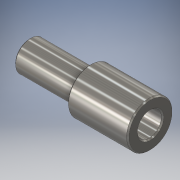
# Autodesk Inventor part: Motor-Adapter
Saved by Autodesk Inventor 2016 (Build 200138000, 138)
## iProperties
Created: 2015-05-19
Part Number: Motor-Adapter
Material: Generic
Document SubType Name: Modeling
Designer: jonathan
Density: 1 g/cm^3
Appearance: Steel - Polished
Mass: 1.0291 g
Surface Area: 9.66443 cm^2
Volume: 1.0291 cm^3
Author: jonathan
Autodesk Inventor part; units mm, degrees
ref_plane "YZ Plane" through (0, 0, 0) normal (1, 0, 0) x (0, 1, 0)
ref_plane "XZ Plane" through (0, 0, 0) normal (0, 1, 0) x (-1, 0, 0)
ref_plane "XY Plane" through (0, 0, 0) normal (0, 0, 1) x (1, 0, 0)
sketch "Sketch1" plane through (0, 0, 0) normal (1, 0, 0) x (0, 1, 0)
  circle A0 centre (0, 0) radius 3.175
  dimension "d0" = 6.35
  constraints: 1 centre point, 1 coincident
  measures "d0" diameter of A0
extrude "Extrusion1" add sketch "Sketch1" along normal blind 12.7
sketch "Sketch2" plane through (12.7, 0, 0) normal (1, 0, 0) x (0, 0, -1)
  circle A0 centre (0, 0) radius 4.7625
  circle A1 centre (0, 0) radius 2.54
  dimension "d3" = 9.525
  dimension "d6" = 5.08
  constraints: 2 centre point, 2 coincident
  measures "d3" diameter of A0
  measures "d6" diameter of A1
extrude "Extrusion2" add sketch "Sketch2" along normal blind 12.7
sketch "Sketch4" plane through (0, 0, 0) normal (0, 1, 0) x (-1, 0, 0)
  circle A0 centre (-15.7257, 0) radius 1.5875
  point P0 (0, 0)
  dimension "d7" = 3.175
  constraints: 1 centre point
  measures "d7" diameter of A0
extrude "Extrusion3" cut sketch "Sketch4" against normal up to next
chamfer "Chamfer1" distance 0.254 angle 45 6 edges at (0, -3.175, 0) (12.7, 0, 4.7625) (12.7, -3.175, 0) (17.2497, -4.7417, 0.4446) (25.4, 0, 4.7625) (25.4, 0, 2.54)
body "Solid1"
